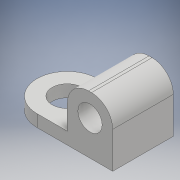
# Autodesk Inventor part: cylinder bracket
Saved by Autodesk Inventor 2017 (Build 210142000, 142)
## iProperties
Created: 2017-12-08
Part Number: cylinder bracket
Material: Generic
Document SubType Name: Modeling
Designer: RLanting
Density: 1 g/cm^3
Appearance: Default
Author: RLanting
Autodesk Inventor part; units mm, degrees
ref_plane "YZ Plane" through (0, 0, 0) normal (1, 0, 0) x (0, 1, 0)
ref_plane "XZ Plane" through (0, 0, 0) normal (0, 1, 0) x (-1, 0, 0)
ref_plane "XY Plane" through (0, 0, 0) normal (0, 0, 1) x (1, 0, 0)
sketch "Sketch1" plane through (0, 0, 0) normal (0, 0, 1) x (1, 0, 0)
  circle A0 centre (0, 0) radius 5
  line L0 (0, 0) -> (25, 0) construction
  line L1 (0, -10) -> (25, -10)
  line L2 (25, 10) -> (0, 10)
  arc A1 (0, 10) -> (0, -10) centre (0, 0) ccw
  arc A2 (25, -10) -> (25, 10) centre (25, 0) ccw construction
  line L3 (25, 10) -> (25, -10)
  point P0 (12.5, 0)
  dimension "d0" = 10
  dimension "d1" = 5
  dimension "d2" = 25
  constraints: 10 end point, 4 point on circle, 4 tangent, 3 centre point, 1 coincident, 1 horizontal, 1 midpoint, 1 parallel, 1 vertical
  measures "d0" diameter of A0
  measures "d1" radial gap between concentric circles of A0 A1
  measures "d2" distance of L0.start L0.end
extrude "Extrusion1" add sketch "Sketch1" along normal blind 4
sketch "Sketch2" plane through (0, -10, 0) normal (0, -1, 0) x (1, 0, 0)
  line L0 (0, 4) -> (25, 4) projected
  line L1 (25, 4) -> (10, 4)
  line L2 (10, 4) -> (10, 19)
  line L3 (10, 19) -> (25, 19)
  line L4 (25, 19) -> (25, 4)
  line L5 (17.5, 19) -> (17.5, 4) construction
  circle A0 centre (17.5, 11.5) radius 4
  point P0 (0, 0)
  dimension "d5" = 8
  dimension "d6" = 15
  dimension "d7" = 15
  constraints: 10 end point, 3 midpoint, 2 parallel, 1 centre point, 1 horizontal, 1 perpendicular
  measures "d5" diameter of A0
  measures "d6" distance of L2.end L3.end
  measures "d7" distance of L3.end L0.end
extrude "Extrusion2" add sketch "Sketch2" against normal up to surface (20 mm away)
fillet "Fillet1" radius 7 2 edges at (25, 0, 19) (10, 0, 19)
body "Solid1"
